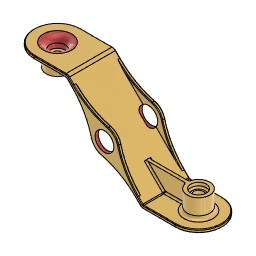
Exercise-22 v1 (Autodesk Fusion 360 design; units mm, degrees)
Autodesk Fusion 360 part; units mm, degrees
sketch "Sketch1" plane through (0, 0, 0) normal (0, 1, 0) x (1, 0, 0)
  circle A0 centre (0, 0) radius 22.5
  circle A1 centre (0, 0) radius 15
  line L0 (0, 0) -> (58.5355, 58.5355) construction
  line L1 (0, 0) -> (72.4273, 0) construction
  line L2 (150, 60) -> (62.0711, 60) construction
  arc A2 (62.0711, 60) -> (58.5355, 58.5355) centre (62.0711, 55) ccw construction
  line L3 (1.7678, -1.7678) -> (60.3033, 56.7678)
  arc A3 (62.0711, 57.5) -> (60.3033, 56.7678) centre (62.0711, 55) ccw
  line L4 (150, 57.5) -> (62.0711, 57.5)
  line L5 (-1.7678, 1.7678) -> (56.7678, 60.3033)
  arc A4 (62.0711, 62.5) -> (56.7678, 60.3033) centre (62.0711, 55) ccw
  line L6 (150, 62.5) -> (62.0711, 62.5)
  line L7 (150, 57.5) -> (150, 62.5)
  arc A5 (53.2459, 49.7104) -> (21.8051, -5.5488) centre (138.0987, -35.1424) ccw
  arc A6 (-5.5488, 21.8051) -> (49.7104, 53.2459) centre (-35.1424, 138.0987) ccw
  arc A7 (-62.0711, -57.5) -> (-60.3033, -56.7678) centre (-62.0711, -55) ccw
  line L8 (-150, -57.5) -> (-150, -62.5)
  arc A8 (-62.0711, -62.5) -> (-56.7678, -60.3033) centre (-62.0711, -55) ccw
  line L9 (0, 0) -> (-58.5355, -58.5355) construction
  arc A9 (5.5488, -21.8051) -> (-49.7104, -53.2459) centre (35.1424, -138.0987) ccw
  line L10 (-150, -60) -> (-62.0711, -60) construction
  line L11 (-150, -62.5) -> (-62.0711, -62.5)
  line L12 (-1.7678, 1.7678) -> (-60.3033, -56.7678)
  line L13 (1.7678, -1.7678) -> (-56.7678, -60.3033)
  arc A10 (-62.0711, -60) -> (-58.5355, -58.5355) centre (-62.0711, -55) ccw construction
  line L14 (-150, -57.5) -> (-62.0711, -57.5)
  arc A11 (-53.2459, -49.7104) -> (-21.8051, 5.5488) centre (-138.0987, 35.1424) ccw
  dimension "d1" = 45
  dimension "d2" = 30
  dimension "d3" = 45
  dimension "d4" = 60
  dimension "d5" = 150
  dimension "d6" = 5
  dimension "d7" = 2.5
  dimension "d8" = -2.5
  dimension "d12" = 5
  constraint coincident A0.centre A1.centre
  constraint horizontal L1
  constraint horizontal L2
  constraint tangent L0 A2
  constraint tangent L2 A2
  constraint perpendicular L6 L7
  constraint coincident A0 A5.end
  constraint coincident L3 A5.start
  constraint symmetric L0 A5.end A6.start
  constraint symmetric L0 A5 A6
  constraint symmetric L0 A5.start A6.end
  constraint tangent L9 A10
  constraint tangent L10 A10
  constraint perpendicular L8 L11
  constraint coincident A11.start L12
  constraint symmetric A9.start A11.end L9
  constraint symmetric L9 A9 A11
  constraint symmetric A9.end A11.start L9
  constraint concentric A7 A10
  constraint tangent A7 L12
  constraint tangent A7 L14
  constraint concentric A8 A10
  constraint tangent A8 L13
  constraint tangent A8 L11
  measures "d1" diameter of A0
  measures "d2" diameter of A1
  measures "d3" angle of L0 L1
  measures "d4" vertical distance of A0.centre L2.start
  measures "d5" horizontal distance of A0.centre L2.start
  measures "d6" radius of A2
  measures "d12" radius of A10
extrude "Extrude1" add sketch "Sketch1" along normal mid plane 75 contours A0 L3 A3 L4 L5 A4 L6 L7 | A0 A1 L3 L5 | A0 A1 L12 L13 | A0 A7 L8 A8 L11 L12 L13 L14 | A1 L3 L5 L12 L13
extrude "Extrude2" cut sketch "Sketch1" along normal blind 15 from surface at 22.5 contours A1 L3 L5 L12 L13
extrude "Extrude3" add sketch "Sketch1" along normal blind 5 from surface at 32.5 contours A0 A1 L5 L12 | A0 A1 L3 L5 | A0 A1 L12 L13 | A0 A1 L3 L13
extrude "Extrude4" add sketch "Sketch1" along normal blind 5 from surface at 32.5 contours A0 L5 A6 | A0 L12 A11 | A0 L3 A5 | A0 A9 L13
fillet "Fillet1" radius 37.5 4 edges at (150, -37.5, -60) (150, 37.5, -60) (-150, -37.5, 60) (-150, 37.5, 60)
fillet "Fillet2" radius 7.5 2 edges at (-10.6066, 22.5, 10.6066) (10.6066, 22.5, -10.6066)
mirror "Mirror1" about plane through (0, 0, 0) normal (0, 1, 0) of "Extrude2", "Extrude3", "Extrude4", "Fillet2"
fillet "Fillet3" radius 1 52 edges at (-56.7746, -37.5, 53.2391) (-61.1144, -37.5, 57.3097) (-87.2855, -37.5, 57.5) (-150, 0, 57.5) (-87.2855, 37.5, 57.5) (-61.1144, 37.5, 57.3097) (-56.7746, 37.5, 53.2391) (-33.7993, 37.5, 24.2009) (-15.9099, 37.5, -15.9099) (24.2009, 37.5, -33.7993) (53.2391, 37.5, -56.7746) (59.2009, 37.5, -61.9291) (87.2855, 37.5, -62.5) (150, 0, -62.5) (87.2855, -37.5, -62.5) (59.2009, -37.5, -61.9291) (53.2391, -37.5, -56.7746) (24.2009, -37.5, -33.7993) (-15.9099, -37.5, -15.9099) (-33.7993, -37.5, 24.2009) (33.7993, -37.5, -24.2009) (56.7746, -37.5, -53.2391) (61.1144, -37.5, -57.3097) (87.2855, -37.5, -57.5) (150, 0, -57.5) (87.2855, 37.5, -57.5) (61.1144, 37.5, -57.3097) (56.7746, 37.5, -53.2391) (33.7993, 37.5, -24.2009) (15.9099, 37.5, 15.9099) (-24.2009, 37.5, 33.7993) (-53.2391, 37.5, 56.7746) (-59.2009, 37.5, 61.9291) (-87.2855, 37.5, 62.5) (-150, 0, 62.5) (-87.2855, -37.5, 62.5) (-59.2009, -37.5, 61.9291) (-53.2391, -37.5, 56.7746) (-24.2009, -37.5, 33.7993) (15.9099, -37.5, 15.9099) (33.7993, -32.5, -24.2009) (15.9099, -32.5, 15.9099) (-24.2009, -32.5, 33.7993) (-24.2009, 32.5, 33.7993) (15.9099, 32.5, 15.9099) (33.7993, 32.5, -24.2009) (24.2009, 32.5, -33.7993) (-15.9099, 32.5, -15.9099) (-33.7993, 32.5, 24.2009) (-33.7993, -32.5, 24.2009) (-15.9099, -32.5, -15.9099) (24.2009, -32.5, -33.7993)
sketch "Sketch2" plane through (0, 0, 62.5) normal (0, 0, 1) x (-1, 0, 0)
  line L0 (62.0711, -36.5) -> (112.5, -36.5)
  arc A0 (112.5, -36.5) -> (112.5, 36.5) centre (112.5, 0) ccw
  line L1 (112.5, 36.5) -> (62.0711, 36.5)
  line L2 (62.0711, 36.5) -> (62.0711, -36.5)
  circle A1 centre (112.5, 0) radius 7.5
  circle A2 centre (112.5, 0) radius 12.5
  circle A3 centre (112.5, 0) radius 18
  dimension "d32" = 15
  dimension "d33" = 25
  dimension "d34" = 36
  constraint concentric A0 A1
  constraint concentric A0 A2
  constraint concentric A2 A3
  measures "d32" diameter of A1
  measures "d33" diameter of A2
  measures "d34" diameter of A3
extrude "Extrude5" add sketch "Sketch2" against normal blind 35 contours A2 | A3
extrude "Extrude6" cut sketch "Sketch2" against normal through all contours A1
extrude "Extrude7" cut sketch "Sketch2" against normal blind 17.5 contours A2
extrude "Extrude8" cut sketch "Sketch2" along normal blind 7.5 from surface at -35 contours A2
fillet "Fillet4" radius 10 1 edges at (-100.8459, -4.5202, 62.5)
fillet "Fillet5" radius 2.5 1 edges at (-100.8459, 4.5202, 35)
fillet "Fillet6" radius 5 1 edges at (-95.7181, 6.5091, 57.5)
sketch "Sketch3" plane through (0, 0, 0) normal (0, 1, 0) x (1, 0, 0)
  line L0 (49.7104, 53.2459) -> (56.7678, 60.3033)
  line L1 (56.7678, 60.3033) -> (49.7104, 53.2459)
  line L2 (49.7104, 53.2459) -> (38.7331, 42.2687)
  line L3 (38.7331, 42.2687) -> (8.6905, 12.226)
  line L4 (3.2322, 6.7678) -> (8.6905, 12.226)
  line L5 (3.2322, 6.7678) -> (-6.7678, -3.2322)
  line L6 (-12.226, -8.6905) -> (-6.7678, -3.2322)
  line L7 (-12.226, -8.6905) -> (-42.2687, -38.7331)
  line L8 (-42.2687, -38.7331) -> (-53.2459, -49.7104)
  line L9 (-53.2459, -49.7104) -> (-60.3033, -56.7678)
  line L10 (-60.3033, -56.7678) -> (-53.2459, -49.7104)
  line L11 (-53.2459, -49.7104) -> (-42.2687, -38.7331)
  line L12 (-42.2687, -38.7331) -> (-12.226, -8.6905)
  line L13 (-6.7678, -3.2322) -> (-12.226, -8.6905)
  line L14 (-6.7678, -3.2322) -> (3.2322, 6.7678)
  line L15 (8.6905, 12.226) -> (3.2322, 6.7678)
  line L16 (8.6905, 12.226) -> (38.7331, 42.2687)
  line L17 (38.7331, 42.2687) -> (49.7104, 53.2459)
  arc A0 (-62.0711, -57.5) -> (-60.3033, -56.7678) centre (-62.0711, -55) ccw
  arc A1 (-62.0711, -57.5) -> (-60.3033, -56.7678) centre (-62.0711, -55) ccw
  line L18 (-112.5, -57.5) -> (-62.0711, -57.5)
  line L19 (-62.0711, -57.5) -> (-112.5, -57.5)
  line L20 (-149, -57.5) -> (-112.5, -57.5)
  line L21 (-89.5, -57.5) -> (-135.5, -57.5)
  line L22 (-94.5, -27.5) -> (-130.5, -27.5)
  line L23 (-89.5, -57.5) -> (-62.0711, -57.5)
  line L24 (-149, -57.5) -> (-135.5, -57.5)
  line L25 (-112.5, -62.5) -> (-149, -62.5)
  line L26 (-62.0711, -62.5) -> (-112.5, -62.5)
  arc A2 (53.2459, 49.7104) -> (21.8051, -5.5488) centre (138.0987, -35.1424) ccw
  line L27 (60.3033, 56.7678) -> (53.2459, 49.7104)
  arc A3 (62.0711, 57.5) -> (60.3033, 56.7678) centre (62.0711, 55) ccw
  line L28 (112.5, 57.5) -> (62.0711, 57.5)
  line L29 (149, 57.5) -> (112.5, 57.5)
  arc A4 (-62.0711, -62.5) -> (-56.7678, -60.3033) centre (-62.0711, -55) ccw
  line L30 (-49.7104, -53.2459) -> (-56.7678, -60.3033)
  arc A5 (5.5488, -21.8051) -> (-49.7104, -53.2459) centre (35.1424, -138.0987) ccw
  arc A6 (5.5488, -21.8051) -> (21.8051, -5.5488) centre (0, 0) ccw
  line L31 (-3.2322, -6.7678) -> (-8.6905, -12.226)
  line L32 (-3.2322, -6.7678) -> (6.7678, 3.2322)
  line L33 (12.226, 8.6905) -> (6.7678, 3.2322)
  line L34 (-60.3033, -56.7678) -> (-53.2459, -49.7104)
  arc A7 (-53.2459, -49.7104) -> (-21.8051, 5.5488) centre (-138.0987, 35.1424) ccw
  arc A8 (-5.5488, 21.8051) -> (-21.8051, 5.5488) centre (0, 0) ccw
  arc A9 (-5.5488, 21.8051) -> (49.7104, 53.2459) centre (-35.1424, 138.0987) ccw
  line L35 (49.7104, 53.2459) -> (56.7678, 60.3033)
  arc A10 (62.0711, 62.5) -> (56.7678, 60.3033) centre (62.0711, 55) ccw
  line L36 (62.0711, 62.5) -> (112.5, 62.5)
  line L37 (112.5, 62.5) -> (149, 62.5)
  arc A11 (-62.0711, -57.5) -> (-60.3033, -56.7678) centre (-62.0711, -55) ccw
  line L38 (3.2322, 6.7678) -> (8.6905, 12.226)
  line L39 (3.2322, 6.7678) -> (-6.7678, -3.2322)
  line L40 (-12.226, -8.6905) -> (-6.7678, -3.2322)
  arc A12 (8.6905, 12.226) -> (-15, 0) centre (0, 0) ccw
  arc A13 (-8.6905, -12.226) -> (12.226, 8.6905) centre (0, 0) ccw
  arc A14 (-15, 0) -> (-12.226, -8.6905) centre (0, 0) ccw
  arc A15 (-94.5, -52.5) -> (-89.5, -57.5) centre (-89.5, -52.5) ccw
  arc A16 (-135.5, -57.5) -> (-130.5, -52.5) centre (-135.5, -52.5) ccw
  line L41 (-94.5, -52.5) -> (-94.5, -27.5)
  line L42 (-130.5, -52.5) -> (-130.5, -27.5)
  arc A17 (149, 57.5) -> (150, 58.5) centre (149, 58.5) ccw
  arc A18 (-150, -61.5) -> (-149, -62.5) centre (-149, -61.5) ccw
  line L43 (150, 61.5) -> (150, 58.5)
  arc A19 (150, 61.5) -> (149, 62.5) centre (149, 61.5) ccw
  arc A20 (-149, -57.5) -> (-150, -58.5) centre (-149, -58.5) ccw
  line L44 (-150, -61.5) -> (-150, -58.5)
  line L45 (-94.5, -27.5) -> (-31.0355, -27.5)
  line L46 (-96, -27.5) -> (-96, -57.5)
  dimension "d49" = 30
  constraint horizontal L45
  constraint coincident L22.start L41.end
  constraint coincident L7 L45.end
  constraint coincident L22 L46.start
  constraint coincident L19 L46.end
  measures "d49" distance of L46.start L46.end
extrude "Extrude9" add sketch "Sketch3" along normal mid plane 5 contours L7 L8 L11 L12 A7 L45 | L9 L10 A0 A1 L18 L19 L23 L34 A7 A11 A15 L41 L45 | L18 L19 L21 L22 A15 L41 L46
fillet "Fillet7" radius 2.5 10 edges at (-45.6694, 2.5, 42.1339) (-61.1144, 2.5, 57.3097) (-75.8537, 2.5, 57.5) (-93.1915, 2.5, 56.0407) (-94.6745, 2.5, 40) (-94.6745, -2.5, 40) (-93.1917, -2.5, 56.0405) (-75.8537, -2.5, 57.5) (-61.1144, -2.5, 57.3097) (-45.6694, -2.5, 42.1339)
pattern_circular "C-Pattern1" count 2 over 360 about axis through (0, 1.75, 0) along (0, 1, 0) of "Extrude5", "Extrude6", "Extrude7", "Extrude8"
fillet "Fillet8" radius 5 1 edges at (95.7181, 6.5091, -57.5)
fillet "Fillet9" radius 2.5 1 edges at (100.8459, 4.5202, -35)
fillet "Fillet10" radius 10 1 edges at (100.8459, -4.5202, -62.5)
pattern_circular "C-Pattern2" count 2 over 360 about axis through (0, 1.75, 0) along (0, 1, 0) of "Extrude9"
fillet "Fillet11" radius 2.5 10 edges at (94.6745, -2.5, -40) (93.1917, -2.5, -56.0405) (75.8537, -2.5, -57.5) (61.1144, -2.5, -57.3097) (45.6694, -2.5, -42.1339) (45.6694, 2.5, -42.1339) (61.1144, 2.5, -57.3097) (75.8537, 2.5, -57.5) (93.1917, 2.5, -56.0405) (94.6745, 2.5, -40)
